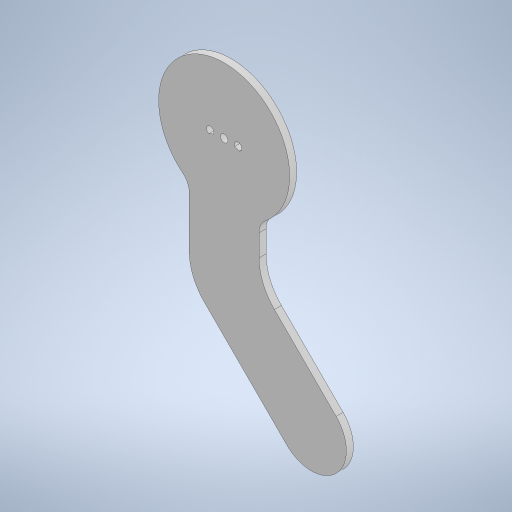
# Autodesk Inventor part: Деталь1
Saved by Autodesk Inventor 2023.1 (Build 271208000, 208)
## iProperties
Created: 2025-10-17
Part Number: Деталь1
Material: Типовые
Document SubType Name: Modeling
Designer: DELL
Density: 1 g/cm^3
Appearance: По умолчанию
Author: DELL
Autodesk Inventor part; units mm, degrees
ref_plane "YZ Plane" through (0, 0, 0) normal (1, 0, 0) x (0, 1, 0)
ref_plane "XZ Plane" through (0, 0, 0) normal (0, 1, 0) x (-1, 0, 0)
ref_plane "XY Plane" through (0, 0, 0) normal (0, 0, 1) x (1, 0, 0)
sketch "Эскиз1" plane through (0, 0, 0) normal (0, 0, 1) x (1, 0, 0)
  circle A0 centre (0, 0) radius 37.5
  circle A1 centre (0, 0) radius 2.1
  circle A2 centre (-8, 0) radius 2.1
  circle A3 centre (8, 0) radius 2.1
  line L0 (0, 0) -> (21.2822, 0) construction
  line L1 (0, 0) -> (-18.9176, 0) construction
  dimension "d0" = 75
  dimension "d1" = 4.2
  dimension "d2" = 4.2
  dimension "d3" = 4.2
  dimension "d4" = 8
  dimension "d5" = 8
  constraints: 4 centre point, 4 end point, 2 coincident, 2 horizontal, 2 point on line
  measures "d0" diameter of A0
  measures "d1" diameter of A1
  measures "d2" diameter of A2
  measures "d3" diameter of A3
  measures "d4" distance of L0.start A3.centre
  measures "d5" distance of L0.start A2.centre
extrude "Выдавливание1" add sketch "Эскиз1" along normal blind 4
sketch "Эскиз2" plane through (0, 0, 4) normal (0, 0, 1) x (1, 0, 0)
  circle A0 centre (0, 0) radius 2.1 projected
  line L0 (0, 0) -> (0, -140) construction
  line L1 (-20, -20) -> (-20, -65.8579)
  arc A1 (20, -20) -> (-20, -20) centre (0, -20) ccw
  line L2 (0, -70) -> (64.1421, -134.1421) construction
  line L3 (0, -98.2843) -> (35.8579, -134.1421)
  line L4 (64.1421, -105.8579) -> (28.2843, -70)
  arc A2 (35.8579, -134.1421) -> (64.1421, -105.8579) centre (50, -120) ccw
  line L5 (0, -70) -> (90.7107, -70) construction
  line L6 (0, -140) -> (114.1632, -140) construction
  line L7 (0, -98.2843) -> (-11.2132, -87.0711)
  arc A3 (-20, -65.8579) -> (-11.2132, -87.0711) centre (10, -65.8579) ccw
  line L8 (28.2843, -70) -> (28.7868, -70.5025)
  line L9 (20, -49.2893) -> (20, -20)
  arc A4 (20, -49.2893) -> (28.7868, -70.5025) centre (50, -49.2893) ccw
  point P0 (32.0711, -102.0711)
  point P1 (2.0971, -0.1103)
  point P2 (-2.0971, -0.1102)
  dimension "d19" = 45
  dimension "d20" = 40
  dimension "d21" = 30
  dimension "d22" = 30
  constraints: 24 end point, 10 point on circle, 9 tangent, 4 centre point, 2 horizontal, 2 midpoint, 2 parallel, 2 point on line, 1 equal length, 1 vertical
  measures "d19" angle of L2 L5
  measures "d20" diameter of A2
  measures "d21" radius of A3
  measures "d22" radius of A4
extrude "Выдавливание2" add sketch "Эскиз2" against normal blind 4 contours A0 A1 L9 A4 L4 A2 L3 L7 A3 L1
fillet "Сопряжение1" radius 10 2 edges at (-20, -31.7214, 2) (20, -31.7214, 2)
